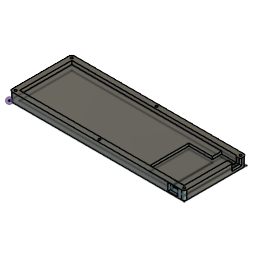
keeb_bottom (Autodesk Fusion 360 archive; units mm, degrees)
design "keeb_bottom" references "RollBoard"
part number: 2026-05-27-19-45-52-835
Autodesk Fusion 360 part; units mm, degrees
sketch "Sketch3" plane through (0, 0, 0) normal (0, 0, 1) x (1, 0, 0)
  line L0 (0, 0) -> (336, 0)
  line L1 (336, 0) -> (336, 120)
  line L2 (336, 120) -> (0, 120)
  line L3 (0, 120) -> (0, 0)
  line L4 (10, 10) -> (326, 10)
  line L5 (326, 10) -> (326, 110)
  line L6 (326, 110) -> (10, 110)
  line L7 (10, 110) -> (10, 10)
  line L8 (326, 110) -> (298, 110)
  line L9 (298, 110) -> (298, 10)
  line L10 (298, 10) -> (326, 10)
  line L11 (326, 10) -> (326, 110)
  line L12 (298, 92) -> (253, 92)
  line L13 (253, 92) -> (253, 17)
  line L14 (253, 17) -> (298, 17)
  line L15 (298, 17) -> (298, 92)
  dimension "d25" = 100
  dimension "d26" = 316
  dimension "d27" = 10
  dimension "d28" = 10
  dimension "d29" = 10
  dimension "d30" = 336
  dimension "d31" = 28
  dimension "d32" = 45
  dimension "d33" = 75
  dimension "d34" = 7
  constraint horizontal L0
  constraint vertical L1
  constraint horizontal L2
  constraint vertical L3
  constraint coincident L0.start L3.end
  constraint horizontal L4
  constraint vertical L5
  constraint horizontal L6
  constraint vertical L7
  constraint horizontal L8
  constraint vertical L9
  constraint horizontal L10
  constraint vertical L11
  constraint horizontal L12
  constraint vertical L13
  constraint horizontal L14
  constraint vertical L15
  constraint coincident L9 L12.start
  measures "d25" distance of L4.start L6.end
  measures "d26" distance of L4.start L4.end
  measures "d27" distance of L2 L6
  measures "d28" distance of L3 L7
  measures "d29" distance of L0 L4
  measures "d30" distance of L0.start L0.end
  measures "d31" distance of L9 L11
  measures "d32" distance of L13.end L14.end
  measures "d33" distance of L12.end L13.end
  measures "d34" distance of L4 L14
extrude "Extrude4" add sketch "Sketch3" along normal blind 5 contours L4 L5 L6 L8 L9 L10 L11 L15 | L9 L12 L13 L14 L15 makes body 1
extrude "Extrude5" add sketch "Sketch3" along normal blind 10 separate body contours L4 L6 L7 L9 L12 L13 L14 makes body 2
extrude "Extrude6" add sketch "Sketch3" along normal blind 17 separate body makes body 3
sketch "Sketch4" plane through (0, 0, 0) normal (0, 0, 1) x (1, 0, 0)
  circle A0 centre (6, 114) radius 2.15
  circle A1 centre (6, 6) radius 2.15
  circle A2 centre (330, 6) radius 2.15
  circle A3 centre (330, 114) radius 2.15
  line L0 (336, 0) -> (336, 120)
  line L1 (336, 120) -> (0, 120)
  line L2 (0, 120) -> (0, 0)
  line L3 (0, 0) -> (336, 0)
  circle A4 centre (168, 5) radius 2.15
  line L4 (10, 10) -> (326, 10)
  circle A5 centre (168, 115) radius 2.15
  dimension "d41" = 4.3
  dimension "d42" = 4.3
  dimension "d43" = 4.3
  dimension "d44" = 4.3
  dimension "d45" = 6
  dimension "d46" = 6
  dimension "d47" = 6
  dimension "d48" = 6
  dimension "d49" = 6
  dimension "d50" = 6
  dimension "d51" = 6
  dimension "d52" = 6
  dimension "d53" = 4.3
  dimension "d54" = 5
  dimension "d55" = 168
  dimension "d56" = 4.3
  dimension "d57" = 5
  dimension "d58" = 168
  measures "d41" diameter of A0
  measures "d42" diameter of A1
  measures "d43" diameter of A2
  measures "d44" diameter of A3
  measures "d45" distance of A3.centre L0
  measures "d46" distance of A3.centre L1
  measures "d47" distance of A0.centre L1
  measures "d48" distance of A0.centre L2
  measures "d49" distance of A1.centre L3
  measures "d50" distance of A1.centre L2
  measures "d51" distance of A2.centre L3
  measures "d52" distance of A2.centre L0
  measures "d53" diameter of A4
  measures "d54" distance of A4.centre L4
  measures "d55" distance of L2 A4.centre
  measures "d56" diameter of A5
  measures "d57" distance of L1 A5.centre
  measures "d58" distance of L2 A5.centre
extrude "Extrude7" cut sketch "Sketch4" along normal blind 17 contours A0 | A1 | A2 | A3 | A4 | A5 bodies 3
extrude "Extrude8" add sketch "Sketch4" along normal blind 11 contours A0 | A1 | A2 | A3 | A4 | A5 bodies 3
sketch "Sketch5" plane through (336, 0, 0) normal (1, 0, 0) x (0, 1, 0)
  line L0 (0, 0) -> (120, 0)
  line L1 (120, 0) -> (120, 17)
  line L2 (120, 17) -> (0, 17)
  line L3 (0, 17) -> (0, 0)
  line L4 (94, 7) -> (108, 7)
  line L5 (108, 7) -> (108, 17)
  line L6 (108, 17) -> (94, 17)
  line L7 (94, 17) -> (94, 7)
  dimension "d63" = 14
  dimension "d64" = 10
  dimension "d65" = 7
  dimension "d66" = 12
  constraint horizontal L4
  constraint vertical L5
  constraint horizontal L6
  constraint vertical L7
  measures "d63" distance of L4.start L4.end
  measures "d64" distance of L4.end L5.end
  measures "d65" distance of L0 L4
  measures "d66" distance of L1 L5
extrude "Extrude9" cut sketch "Sketch5" against normal blind 10 contours L2 L4 L5 L6 L7 bodies 3
fillet "Fillet5" radius 2.5 1 edges at (336, 108, 12) on bodies 3
fillet "Fillet6" radius 2.5 1 edges at (336, 102.25, 7) on bodies 3
fillet "Fillet7" radius 2.5 1 edges at (336, 94, 10.75) on bodies 3
fillet "Fillet8" radius 5 1 edges at (336, 120, 8.5) on bodies 3
fillet "Fillet9" radius 2.5 1 edges at (326, 108, 12) on bodies 3
fillet "Fillet10" radius 2.5 1 edges at (326, 102, 7) on bodies 3
fillet "Fillet11" radius 2.5 1 edges at (326, 94, 10.75) on bodies 3
sketch "Sketch6" plane through (0, 0, 0) normal (0, 1, 0) x (1, 0, 0)
  line L0 (321, -4) -> (307, -4)
  line L1 (307, -4) -> (307, -14)
  line L2 (307, -14) -> (321, -14)
  line L3 (321, -14) -> (321, -4)
  line L4 (336, 0) -> (336, -17)
  line L5 (0, -17) -> (336, -17)
  dimension "d83" = 15
  dimension "d84" = 14
  dimension "d85" = 10
  dimension "d86" = 3
  constraint horizontal L0
  constraint vertical L1
  constraint horizontal L2
  constraint vertical L3
  measures "d83" distance of L3 L4
  measures "d84" distance of L1.end L2.end
  measures "d85" distance of L0.end L1.end
  measures "d86" distance of L2 L5
extrude "Extrude10" cut sketch "Sketch6" along normal blind 10 bodies 3
fillet "Fillet12" radius 2.5 4 edges at (314, 0, 4) (307, 0, 9) (321, 0, 9) (314, 0, 14) on bodies 3
fillet "Fillet13" radius 2.5 3 edges at (314, 10, 14) (321, 10, 9) (307, 10, 9) on bodies 3
fillet "Fillet14" radius 2.5 1 edges at (312, 10, 5) on bodies 1
fillet "Fillet15" radius 5 1 edges at (336, 0, 8.5) on bodies 3
fillet "Fillet16" radius 5 1 edges at (0, 0, 8.5) on bodies 3
fillet "Fillet17" radius 5 1 edges at (0, 120, 8.5) on bodies 3
sketch "Sketch1" plane through (0, 0, 0) normal (0, 0, 1) x (1, 0, 0)
  line L0 (0, 0) -> (326, 0)
  line L1 (326, 0) -> (326, 110)
  line L2 (326, 110) -> (0, 110)
  line L3 (0, 110) -> (0, 0)
  line L4 (5, 5) -> (321, 5)
  line L5 (321, 5) -> (321, 105)
  line L6 (321, 105) -> (5, 105)
  line L7 (5, 105) -> (5, 5)
  line L8 (5, 105) -> (293, 105)
  line L9 (293, 105) -> (293, 5.2328)
  line L10 (293, 5.2328) -> (5, 5.2328)
  line L11 (5, 5.2328) -> (5, 105)
  line L12 (293, 11.7328) -> (248, 11.7328)
  line L13 (248, 11.7328) -> (248, 86.7328)
  line L14 (248, 86.7328) -> (293, 86.7328)
  line L15 (293, 86.7328) -> (293, 11.7328)
  dimension "d1" = 110
  dimension "d2" = 326
  dimension "d3" = 5
  dimension "d4" = 5
  dimension "d5" = 5
  dimension "d6" = 5
  dimension "d7" = 28
  dimension "d8" = 75
  dimension "d9" = 45
  dimension "d10" = 6.5
  constraint horizontal L0
  constraint vertical L1
  constraint horizontal L2
  constraint vertical L3
  constraint coincident L0.start L3.end
  constraint horizontal L4
  constraint vertical L5
  constraint horizontal L6
  constraint vertical L7
  constraint horizontal L8
  constraint vertical L9
  constraint horizontal L10
  constraint vertical L11
  constraint horizontal L12
  constraint vertical L13
  constraint horizontal L14
  constraint vertical L15
  constraint coincident L9 L12.start
  measures "d1" distance of L0.start L2.end
  measures "d2" distance of L0.start L0.end
  measures "d3" distance of L3 L7
  measures "d4" distance of L2 L6
  measures "d5" distance of L0 L4
  measures "d6" distance of L1 L5
  measures "d7" distance of L5 L9
  measures "d8" distance of L12.end L13.end
  measures "d9" distance of L12.start L12.end
  measures "d10" distance of L10 L12
extrude "Extrude1" [suppressed]
extrude "Extrude2" [suppressed]
extrude "Extrude3" [suppressed]
fillet "Fillet1" [suppressed]
fillet "Fillet2" [suppressed]
fillet "Fillet3" [suppressed]
fillet "Fillet4" [suppressed]
sketch "Sketch2" plane through (0, 0, 15) normal (0, 0, 1) x (-1, 0, 0)
  line L0 (-293, -11.7328) -> (-248, -11.7328)
  line L1 (-248, -11.7328) -> (-248, -86.7328)
  line L2 (-248, -86.7328) -> (-293, -86.7328)
  line L3 (-293, -86.7328) -> (-293, -105)
  line L4 (-293, -105) -> (-5, -105)
  line L5 (-5, -105) -> (-5, -5.2328)
  line L6 (-5, -5.2328) -> (-293, -5.2328)
  line L7 (-293, -5.2328) -> (-293, -11.7328)
